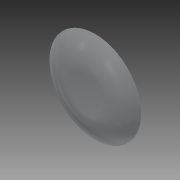
# Autodesk Inventor part: lensGlass
Saved by Autodesk Inventor 2013 (Build 170138000, 138)
## iProperties
Created: 2014-07-04
Part Number: lensGlass
Material: Glass
Document SubType Name: Modeling
Designer: Nano
Mass: 4.76977 g
Surface Area: 18.1775 cm^2
Volume: 2.18797 cm^3
Density: 2.18 g/cm^3
Author: Nano
Autodesk Inventor part; units mm, degrees
ref_plane "YZ Plane" through (0, 0, 0) normal (1, 0, 0) x (0, 1, 0)
ref_plane "XZ Plane" through (0, 0, 0) normal (0, 1, 0) x (-1, 0, 0)
ref_plane "XY Plane" through (0, 0, 0) normal (0, 0, 1) x (1, 0, 0)
sketch "Sketch1" plane through (0, 0, 0) normal (0, 0, 1) x (1, 0, 0)
  circle A0 centre (0, 0) radius 16.6314
  constraints: 1 centre point
extrude "Extrusion1" add sketch "Sketch1" along normal blind 3.81
fillet "Fillet1" radius 16.51 1 edges at (-16.6314, 0, 3.81)
body "Solid1"
